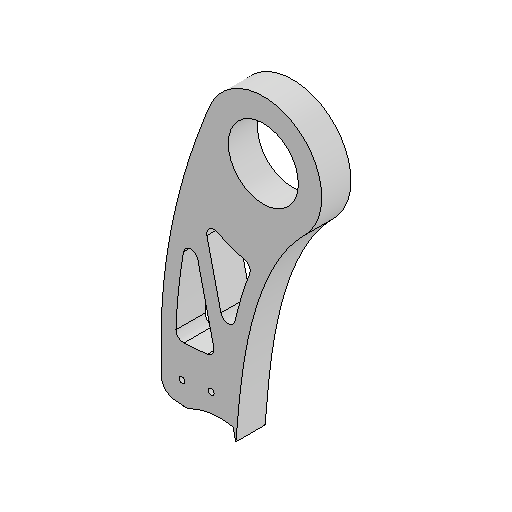
# Autodesk Inventor part: driveshaftsupport_A
Saved by Autodesk Inventor 2025 (Build 290162000, 162)
## iProperties
Created: 2023-03-01
Part Number: driveshaftsupport_A
Material: Generic
Document SubType Name: Modeling
Designer: ralph
Density: 1 g/cm^3
Appearance: Default
Author: ralph
Autodesk Inventor part; units mm, degrees
(part 1 of 2)
ref_plane "YZ Plane" through (0, 0, 0) normal (1, 0, 0) x (0, 1, 0)
ref_plane "XZ Plane" through (0, 0, 0) normal (0, 1, 0) x (-1, 0, 0)
ref_plane "XY Plane" through (0, 0, 0) normal (0, 0, 1) x (1, 0, 0)
ref_plane "Work Plane1" through (0, 0, 0) normal (0, 0, 1) x (1, 0, 0)
sketch "Sketch1" plane through (0, 0, 0) normal (0, 0, 1) x (1, 0, 0)
  arc A0 (-20.648, -102.4649) -> (-16.3515, -107.2084) centre (-14.4346, -101.1546) ccw
  arc A1 (-10.9828, -109.2489) -> (-16.3515, -107.2084) centre (-31.6865, -155.6385) ccw
  arc A2 (-10.9828, -109.2489) -> (-4.2979, -108.3017) centre (-8.3948, -103.4502) ccw
  arc A3 (0.8876, -104.599) -> (-4.2979, -108.3017) centre (21.0506, -138.319) ccw
  arc A4 (7.2668, -104.5186) -> (0.8876, -104.599) centre (4.1465, -110.049) ccw
  arc A5 (7.2668, -104.5186) -> (24.5776, -101.9869) centre (14.2875, -92.075) ccw
  arc A6 (30.7127, -100.2372) -> (24.5776, -101.9869) centre (29.151, -106.3922) ccw
  arc A7 (43.0033, -105.7359) -> (30.7127, -100.2372) centre (21.0506, -138.319) ccw
  arc A8 (43.0033, -105.7359) -> (57.752, -89.4091) centre (49.2125, -96.52) ccw
  arc A9 (57.752, -7.1109) -> (57.752, -89.4091) centre (107.1678, -48.26) ccw
  arc A10 (57.752, -7.1109) -> (57.752, 7.1109) centre (49.2125, 0) ccw
  arc A11 (57.752, 89.4091) -> (57.752, 7.1109) centre (107.1678, 48.26) ccw
  arc A12 (57.752, 89.4091) -> (46.7209, 107.3496) centre (49.2125, 96.52) ccw
  arc A13 (37.2777, 118.8104) -> (46.7209, 107.3496) centre (44.8601, 115.4372) ccw
  arc A14 (37.2777, 118.8104) -> (27.7131, 132.1679) centre (28.575, 122.682) ccw
  arc A15 (-1.8719, 154.7102) -> (27.7131, 132.1679) centre (25.2222, 159.584) ccw
  arc A16 (-1.8719, 154.7102) -> (-9.0898, 161.7077) centre (-11.1125, 152.4) ccw
  arc A17 (-57.3497, 188.5663) -> (-9.0898, 161.7077) centre (11.1567, 254.8735) ccw
  arc A18 (-57.3497, 188.5663) -> (-61.9125, 190.5) centre (-61.9125, 184.15) ccw
  line L0 (-61.9125, -74.837) -> (-61.9125, 190.5)
  arc A19 (-57.4675, -76.6522) -> (-61.9125, -74.837) centre (-61.9125, -81.187) ccw
  arc A20 (-57.4675, -76.6522) -> (-50.3955, -79.3664) centre (-50.8, -69.85) ccw
  arc A21 (-20.648, -102.4649) -> (-50.3955, -79.3664) centre (-49.1581, -108.4774) ccw
  line L1 (-54.9779, 170.3652) -> (-48.8256, 159.5987)
  arc A22 (-48.8539, 153.2488) -> (-48.8256, 159.5987) centre (-54.339, 156.4482) ccw
  arc A23 (-48.8539, 153.2488) -> (-49.1732, 139.4288) centre (-36.5125, 146.05) ccw
  arc A24 (-49.4382, 133.0844) -> (-49.1732, 139.4288) centre (-54.8001, 136.4861) ccw
  line L2 (-49.4382, 133.0844) -> (-55.0158, 124.2927)
  arc A25 (-57.9437, 125.1431) -> (-55.0158, 124.2927) centre (-56.3562, 125.1431) ccw
  line L3 (-57.9437, 125.1431) -> (-57.9437, 169.5776)
  arc A26 (-54.9779, 170.3652) -> (-57.9437, 169.5776) centre (-56.3562, 169.5776) ccw
  line L4 (-57.9437, 16.3803) -> (-57.9437, 88.2093)
  arc A27 (-48.4371, 93.7191) -> (-57.9437, 88.2093) centre (-51.5937, 88.2093) ccw
  line L5 (-48.4371, 93.7191) -> (25.1122, 51.5817)
  arc A28 (24.9048, 45.9631) -> (25.1122, 51.5817) centre (23.5339, 48.8268) ccw
  line L6 (24.9048, 45.9631) -> (-48.8518, 10.6528)
  arc A29 (-57.9437, 16.3803) -> (-48.8518, 10.6528) centre (-51.5937, 16.3803) ccw
  line L7 (-12.5571, -63.0775) -> (-11.8021, -62.3567)
  arc A30 (-6.8531, -63.0782) -> (-11.8021, -62.3567) centre (-9.6098, -64.6534) ccw
  line L8 (-6.8531, -63.0782) -> (0.9035, -76.6523)
  arc A31 (-1.2505, -78.8251) -> (0.9035, -76.6523) centre (-0.4748, -77.44) ccw
  line L9 (-1.2505, -78.8251) -> (-11.2752, -73.2112)
  arc A32 (-12.5571, -63.0775) -> (-11.2752, -73.2112) centre (-8.1726, -67.6708) ccw
  line L10 (8.063, -43.7132) -> (40.1759, -13.8303)
  arc A33 (42.6746, -15.7078) -> (40.1759, -13.8303) centre (41.2574, -14.9925) ccw
  arc A34 (42.6746, -15.7078) -> (35.0956, -43.2986) centre (107.1678, -48.26) ccw
  arc A35 (28.7606, -49.2125) -> (35.0956, -43.2986) centre (28.7606, -42.8625) ccw
  line L11 (28.7606, -49.2125) -> (10.2259, -49.2125)
  arc A36 (8.063, -43.7132) -> (10.2259, -49.2125) centre (10.2259, -46.0375) ccw
  arc A37 (0.0566, -90.8047) -> (0.0035, -91.7596) centre (14.2875, -92.075) ccw
  arc A38 (-5.1562, -94.1671) -> (0.0035, -91.7596) centre (-3.1707, -91.6895) ccw
  arc A39 (-5.1562, -94.1671) -> (-8.4369, -92.4585) centre (-11.1125, -101.6) ccw
  arc A40 (-12.4439, -88.97) -> (-8.4369, -92.4585) centre (-6.6532, -86.3642) ccw
  line L12 (-12.4439, -88.97) -> (-14.871, -83.5766)
  arc A41 (-12.6476, -81.54) -> (-14.871, -83.5766) centre (-13.4233, -82.9251) ccw
  line L13 (-12.6476, -81.54) -> (-1.5545, -87.7521)
  arc A42 (0.0566, -90.8047) -> (-1.5545, -87.7521) centre (-3.1058, -90.5224) ccw
  line L14 (35.1248, 3.9688) -> (-30.4467, 3.9688)
  arc A43 (-31.8177, 10.0075) -> (-30.4467, 3.9688) centre (-30.4467, 7.1438) ccw
  line L15 (-31.8177, 10.0075) -> (27.4027, 38.3586)
  arc A44 (36.3678, 33.8939) -> (27.4027, 38.3586) centre (30.1446, 32.6312) ccw
  arc A45 (36.3678, 33.8939) -> (42.7868, 15.4863) centre (107.1678, 48.26) ccw
  arc A46 (41.5223, 8.0217) -> (42.7868, 15.4863) centre (37.1279, 12.6056) ccw
  arc A47 (41.5223, 8.0217) -> (40.2476, 6.5665) centre (49.2125, 0) ccw
  arc A48 (35.1248, 3.9688) -> (40.2476, 6.5665) centre (35.1248, 10.3188) ccw
  line L16 (-30.2893, 128.8322) -> (-21.4237, 114.8579)
  arc A49 (-24.1047, 109.982) -> (-21.4237, 114.8579) centre (-24.1047, 113.157) ccw
  line L17 (-24.1047, 109.982) -> (-43.146, 109.982)
  arc A50 (-48.5079, 119.7337) -> (-43.146, 109.982) centre (-43.146, 116.332) ccw
  line L18 (-48.5079, 119.7337) -> (-42.7357, 128.8322)
  arc A51 (-37.1087, 131.7749) -> (-42.7357, 128.8322) centre (-37.3737, 125.4305) ccw
  arc A52 (-37.1087, 131.7749) -> (-35.9163, 131.7749) centre (-36.5125, 146.05) ccw
  arc A53 (-30.2893, 128.8322) -> (-35.9163, 131.7749) centre (-35.6513, 125.4305) ccw
  arc A54 (-26.2357, 155.9757) -> (-36.4489, 160.3374) centre (-36.5125, 146.05) ccw
  arc A55 (-41.934, 163.5368) -> (-36.4489, 160.3374) centre (-36.4206, 166.6873) ccw
  line L19 (-41.934, 163.5368) -> (-43.2662, 165.8683)
  arc A56 (-41.0698, 168.0164) -> (-43.2662, 165.8683) centre (-41.8879, 166.6559) ccw
  arc A57 (-41.0698, 168.0164) -> (-20.6642, 158.6488) centre (11.1567, 254.8735) ccw
  arc A58 (-19.7269, 156.4642) -> (-20.6642, 158.6488) centre (-21.1626, 157.1416) ccw
  arc A59 (-19.7269, 156.4642) -> (-20.2275, 155.1645) centre (-11.1125, 152.4) ccw
  arc A60 (-21.7728, 154.038) -> (-20.2275, 155.1645) centre (-21.7467, 155.6253) ccw
  arc A61 (-26.2357, 155.9757) -> (-21.7728, 154.038) centre (-21.6682, 160.3871) ccw
  arc A62 (39.7212, 90.7404) -> (41.5223, 88.4983) centre (49.2125, 96.52) ccw
  arc A63 (42.7868, 81.0337) -> (41.5223, 88.4983) centre (37.1279, 83.9144) ccw
  arc A64 (42.7868, 81.0337) -> (36.5882, 63.6726) centre (107.1678, 48.26) ccw
  arc A65 (27.2278, 59.5175) -> (36.5882, 63.6726) centre (30.3844, 65.0273) ccw
  line L20 (27.2278, 59.5175) -> (-38.1265, 96.9599)
  arc A66 (-37.2022, 99.9191) -> (-38.1265, 96.9599) centre (-37.3374, 98.3373) ccw
  line L21 (-37.2022, 99.9191) -> (34.8381, 93.7648)
  arc A67 (39.7212, 90.7404) -> (34.8381, 93.7648) centre (34.2976, 87.4378) ccw
  line L22 (-57.9437, -42.8625) -> (-57.9437, -24.653)
  arc A68 (-47.137, -20.1298) -> (-57.9437, -24.653) centre (-51.5937, -24.653) ccw
  line L23 (-47.137, -20.1298) -> (-23.138, -43.7759)
  arc A69 (-25.3663, -49.2125) -> (-23.138, -43.7759) centre (-25.3663, -46.0375) ccw
  line L24 (-25.3663, -49.2125) -> (-51.5937, -49.2125)
  arc A70 (-57.9437, -42.8625) -> (-51.5937, -49.2125) centre (-51.5937, -42.8625) ccw
  arc A71 (33.2333, -92.6915) -> (32.5694, -92.5194) centre (21.0506, -138.319) ccw
  arc A72 (28.0165, -88.1193) -> (32.5694, -92.5194) centre (34.1183, -86.3612) ccw
  arc A73 (28.0165, -88.1193) -> (26.6289, -84.8762) centre (14.2875, -92.075) ccw
  arc A74 (26.6006, -78.5263) -> (26.6289, -84.8762) centre (32.114, -81.6768) ccw
  line L25 (26.6006, -78.5263) -> (34.1483, -65.3178)
  arc A75 (37.0671, -65.7217) -> (34.1483, -65.3178) centre (35.5267, -66.1055) ccw
  arc A76 (37.0671, -65.7217) -> (42.7868, -81.0337) centre (107.1678, -48.26) ccw
  arc A77 (41.5223, -88.4983) -> (42.7868, -81.0337) centre (37.1279, -83.9144) ccw
  arc A78 (41.5223, -88.4983) -> (40.0864, -90.1796) centre (49.2125, -96.52) ccw
  arc A79 (33.2333, -92.6915) -> (40.0864, -90.1796) centre (34.8714, -86.5564) ccw
  line L26 (26.9592, -61.9002) -> (19.8008, -74.4274)
  arc A80 (8.7742, -74.4274) -> (19.8008, -74.4274) centre (14.2875, -71.2769) ccw
  line L27 (8.7742, -74.4274) -> (4.3302, -66.6505)
  arc A81 (9.8436, -57.15) -> (4.3302, -66.6505) centre (9.8436, -63.5) ccw
  line L28 (9.8436, -57.15) -> (24.2025, -57.15)
  arc A82 (26.9592, -61.9002) -> (24.2025, -57.15) centre (24.2025, -60.325) ccw
  line L29 (-36.7375, -3.9687) -> (31.0491, -3.9688)
  arc A83 (33.212, -9.4681) -> (31.0491, -3.9688) centre (31.0491, -7.1437) ccw
  line L30 (33.212, -9.4681) -> (-3.4078, -43.5448)
  arc A84 (-12.1903, -43.4194) -> (-3.4078, -43.5448) centre (-7.7336, -38.8962) ccw
  line L31 (-12.1903, -43.4194) -> (-41.1943, -14.842)
  arc A85 (-36.7375, -3.9687) -> (-41.1943, -14.842) centre (-36.7375, -10.3187) ccw
  arc A86 (-23.8518, 139.4288) -> (-22.4829, 143.3475) centre (-36.5125, 146.05) ccw
  arc A87 (-17.3021, 145.1602) -> (-22.4829, 143.3475) centre (-19.3652, 142.7469) ccw
  arc A88 (-17.3021, 145.1602) -> (-16.4703, 144.5248) centre (-11.1125, 152.4) ccw
  arc A89 (-15.0812, 141.8997) -> (-16.4703, 144.5248) centre (-18.2562, 141.8997) ccw
  line L32 (-15.0812, 141.8997) -> (-15.0812, 125.1431)
  arc A90 (-18.0092, 124.2927) -> (-15.0812, 125.1431) centre (-16.6687, 125.1431) ccw
  line L33 (-18.0092, 124.2927) -> (-23.5868, 133.0844)
  arc A91 (-23.8518, 139.4288) -> (-23.5868, 133.0844) centre (-18.2249, 136.4861) ccw
  circle A92 centre (-11.1125, -101.6) radius 3.175
  circle A93 centre (-11.1125, 152.4) radius 3.175
  circle A94 centre (-50.8, -69.85) radius 3.175
  circle A95 centre (-36.5125, 146.05) radius 7.9375
  circle A96 centre (14.2875, -92.075) radius 7.9375
  circle A97 centre (49.2125, 96.52) radius 3.175
  circle A98 centre (49.2125, 0) radius 3.175
  circle A99 centre (49.2125, -96.52) radius 3.175
  circle A100 centre (3.175, 122.682) radius 3.175
  circle A101 centre (-25.4, -69.85) radius 3.175
  circle A102 centre (28.575, 122.682) radius 3.175
  circle A103 centre (-17.4625, 279.4) radius 15.9004
  circle A104 centre (6.6997, 203.792) radius 13.97
  arc A105 (-21.0789, 185.9407) -> (-20.5213, 185.1014) centre (6.6997, 203.792) ccw
  arc A106 (-20.5213, 185.1014) -> (-17.7421, 186.0963) centre (-23.3828, 197.4749) ccw
  arc A107 (-17.7421, 186.0963) -> (-16.917, 185.0092) centre (6.6997, 203.792) ccw
  arc A108 (-16.917, 185.0092) -> (-18.6225, 182.5999) centre (-7.4744, 176.5163) ccw
  arc A109 (-18.6225, 182.5999) -> (-17.9641, 181.8371) centre (6.6997, 203.792) ccw
  arc A110 (-17.9641, 181.8371) -> (-15.3315, 183.1724) centre (-22.3539, 193.7543) ccw
  arc A111 (-15.3315, 183.1724) -> (-14.3766, 182.1973) centre (6.6997, 203.792) ccw
  arc A112 (-14.3766, 182.1973) -> (-15.7668, 179.5933) centre (-3.9441, 174.9549) ccw
  arc A113 (-15.7668, 179.5933) -> (-15.018, 178.919) centre (6.6997, 203.792) ccw
  arc A114 (-15.018, 178.919) -> (-12.5735, 180.5738) centre (-20.8667, 190.1921) ccw
  arc A115 (-12.5735, 180.5738) -> (-11.5039, 179.726) centre (6.6997, 203.792) ccw
  arc A116 (-11.5039, 179.726) -> (-12.5567, 176.9683) centre (-0.246, 173.8483) ccw
  arc A117 (-12.5567, 176.9683) -> (-11.7293, 176.3932) centre (6.6997, 203.792) ccw
  arc A118 (-11.7293, 176.3932) -> (-9.5115, 178.3413) centre (-18.9448, 186.8443) ccw
  arc A119 (-9.5115, 178.3413) -> (-8.3441, 177.6343) centre (6.6997, 203.792) ccw
  arc A120 (-8.3441, 177.6343) -> (-9.043, 174.7663) centre (3.5618, 173.2139) ccw
  arc A121 (-9.043, 174.7663) -> (-8.15, 174.2995) centre (6.6997, 203.792) ccw
  arc A122 (-8.15, 174.2995) -> (-6.1939, 176.5101) centre (-16.6185, 183.7639) ccw
  arc A123 (-6.1939, 176.5101) -> (-4.9471, 175.955) centre (6.6997, 203.792) ccw
  arc A124 (-4.9471, 175.955) -> (-5.281, 173.0221) centre (7.4189, 173.0617) ccw
  arc A125 (-5.281, 173.0221) -> (-4.3365, 172.6709) centre (6.6997, 203.792) ccw
  arc A126 (-4.3365, 172.6709) -> (-2.6729, 175.1093) centre (-13.9245, 180.9992) ccw
  arc A127 (-2.6729, 175.1093) -> (-1.3663, 174.7148) centre (6.6997, 203.792) ccw
  arc A128 (-1.3663, 174.7148) -> (-1.33, 171.7632) centre (11.2648, 173.3941) ccw
  arc A129 (-1.33, 171.7632) -> (-0.349, 171.5331) centre (6.6997, 203.792) ccw
  arc A130 (-0.349, 171.5331) -> (0.9959, 174.1607) centre (-10.9052, 178.5941) ccw
  arc A131 (0.9959, 174.1607) -> (2.3416, 173.9331) centre (6.6997, 203.792) ccw
  arc A132 (2.3416, 173.9331) -> (2.7476, 171.0093) centre (15.0387, 174.206) ccw
  arc A133 (2.7476, 171.0093) -> (3.7497, 170.904) centre (6.6997, 203.792) ccw
  arc A134 (3.7497, 170.904) -> (4.7547, 173.6795) centre (-7.6082, 176.5863) ccw
  arc A135 (4.7547, 173.6795) -> (6.1183, 173.6224) centre (6.6997, 203.792) ccw
  arc A136 (6.1183, 173.6224) -> (6.8875, 170.7725) centre (18.681, 175.4844) ccw
  arc A137 (6.8875, 170.7725) -> (7.8949, 170.7936) centre (6.6997, 203.792) ccw
  arc A138 (7.8949, 170.7936) -> (8.5441, 173.6732) centre (-4.0856, 175.0075) ccw
  arc A139 (8.5441, 173.6732) -> (9.9041, 173.7874) centre (6.6997, 203.792) ccw
  arc A140 (9.9041, 173.7874) -> (11.0244, 171.0564) centre (22.1344, 177.2093) ccw
  arc A141 (11.0244, 171.0564) -> (12.0213, 171.2036) centre (6.6997, 203.792) ccw
  arc A142 (12.0213, 171.2036) -> (12.3044, 174.1418) centre (-0.3929, 173.8827) ccw
  arc A143 (12.3044, 174.1418) -> (13.6394, 174.4256) centre (6.6997, 203.792) ccw
  arc A144 (13.6394, 174.4256) -> (15.0932, 171.8565) centre (25.3444, 179.3534) ccw
  arc A145 (15.0932, 171.8565) -> (16.0637, 172.1275) centre (6.6997, 203.792) ccw
  arc A146 (16.0637, 172.1275) -> (15.9764, 175.0781) centre (3.4116, 173.2296) ccw
  arc A147 (15.9764, 175.0781) -> (17.2653, 175.5269) centre (6.6997, 203.792) ccw
  arc A148 (17.2653, 175.5269) -> (19.0296, 173.1603) centre (28.2603, 181.8829) ccw
  arc A149 (19.0296, 173.1603) -> (19.9585, 173.5508) centre (6.6997, 203.792) ccw
  arc A150 (19.9585, 173.5508) -> (19.502, 176.4672) centre (7.268, 173.0585) ccw
  arc A151 (19.502, 176.4672) -> (20.7245, 177.074) centre (6.6997, 203.792) ccw
  arc A152 (20.7245, 177.074) -> (22.7715, 174.9472) centre (30.8363, 184.7579) ccw
  arc A153 (22.7715, 174.9472) -> (23.6442, 175.451) centre (6.6997, 203.792) ccw
  arc A154 (23.6442, 175.451) -> (22.8258, 178.2872) centre (11.1155, 173.3721) ccw
  arc A155 (22.8258, 178.2872) -> (23.9626, 179.0424) centre (6.6997, 203.792) ccw
  arc A156 (23.9626, 179.0424) -> (26.26, 177.189) centre (33.0315, 187.9331) ccw
  arc A157 (26.26, 177.189) -> (27.0626, 177.7982) centre (6.6997, 203.792) ccw
  arc A158 (27.0626, 177.7982) -> (25.8952, 180.5094) centre (14.8933, 174.1654) ccw
  arc A159 (25.8952, 180.5094) -> (26.9284, 181.4012) centre (6.6997, 203.792) ccw
  arc A160 (26.9284, 181.4012) -> (29.44, 179.8503) centre (34.8116, 191.3584) ccw
  arc A161 (29.44, 179.8503) -> (30.1599, 180.5553) centre (6.6997, 203.792) ccw
  arc A162 (30.1599, 180.5553) -> (28.6619, 183.0989) centre (18.5419, 175.4259) ccw
  arc A163 (28.6619, 183.0989) -> (29.5752, 184.1131) centre (6.6997, 203.792) ccw
  arc A164 (29.5752, 184.1131) -> (32.2613, 182.8892) centre (36.1482, 194.9798) ccw
  arc A165 (32.2613, 182.8892) -> (32.8872, 183.6789) centre (6.6997, 203.792) ccw
  arc A166 (32.8872, 183.6789) -> (31.0823, 186.0146) centre (22.0037, 177.1338) ccw
  arc A167 (31.0823, 186.0146) -> (31.8612, 187.1353) centre (6.6997, 203.792) ccw
  arc A168 (31.8612, 187.1353) -> (34.6796, 186.2577) centre (37.0205, 198.7401) ccw
  arc A169 (34.6796, 186.2577) -> (35.2016, 187.1197) centre (6.6997, 203.792) ccw
  arc A170 (35.2016, 187.1197) -> (33.1181, 189.2107) centre (25.2242, 179.2621) ccw
  arc A171 (33.1181, 189.2107) -> (33.7504, 190.4202) centre (6.6997, 203.792) ccw
  arc A172 (33.7504, 190.4202) -> (36.6566, 189.9028) centre (37.4145, 202.5802) ccw
  arc A173 (36.6566, 189.9028) -> (37.0664, 190.8233) centre (6.6997, 203.792) ccw
  arc A174 (37.0664, 190.8233) -> (34.7373, 192.6368) centre (28.1525, 181.7773) ccw
  arc A175 (34.7373, 192.6368) -> (35.2131, 193.916) centre (6.6997, 203.792) ccw
  arc A176 (35.2131, 193.916) -> (38.1611, 193.7669) centre (37.3242, 206.4393) ccw
  arc A177 (38.1611, 193.7669) -> (38.4524, 194.7316) centre (6.6997, 203.792) ccw
  arc A178 (38.4524, 194.7316) -> (35.9143, 196.2388) centre (30.7425, 184.6396) ccw
  arc A179 (35.9143, 196.2388) -> (36.226, 197.5675) centre (6.6997, 203.792) ccw
  arc A180 (36.226, 197.5675) -> (39.1695, 197.7891) centre (36.7509, 210.2567) ccw
  arc A181 (39.1695, 197.7891) -> (39.3376, 198.7827) centre (6.6997, 203.792) ccw
  arc A182 (39.3376, 198.7827) -> (36.6306, 199.9599) centre (32.9533, 187.804) ccw
  arc A183 (36.6306, 199.9599) -> (36.7733, 201.3172) centre (6.6997, 203.792) ccw
  arc A184 (36.7733, 201.3172) -> (39.6658, 201.906) centre (35.7037, 213.9721) ccw
  arc A185 (39.6658, 201.906) -> (39.708, 202.9128) centre (6.6997, 203.792) ccw
  arc A186 (39.708, 202.9128) -> (36.8749, 203.7415) centre (34.7502, 191.2205) ccw
  arc A187 (36.8749, 203.7415) -> (36.8463, 205.106) centre (6.6997, 203.792) ccw
  arc A188 (36.8463, 205.106) -> (39.6423, 206.0526) centre (34.1991, 217.527) ccw
  arc A189 (39.6423, 206.0526) -> (39.558, 207.0567) centre (6.6997, 203.792) ccw
  arc A190 (39.558, 207.0567) -> (36.6433, 207.5238) centre (36.1046, 194.8353) ccw
  arc A191 (36.6433, 207.5238) -> (36.4439, 208.874) centre (6.6997, 203.792) ccw
  arc A192 (36.4439, 208.874) -> (39.0992, 210.1636) centre (32.2608, 220.8653) ccw
  arc A193 (39.0992, 210.1636) -> (38.8897, 211.1492) centre (6.6997, 203.792) ccw
  arc A194 (38.8897, 211.1492) -> (35.9394, 211.2473) centre (36.9953, 198.5913) ccw
  arc A195 (35.9394, 211.2473) -> (35.5724, 212.5618) centre (6.6997, 203.792) ccw
  arc A196 (35.5724, 212.5618) -> (38.0451, 214.1741) centre (29.9194, 223.9343) ccw
  arc A197 (38.0451, 214.1741) -> (37.7137, 215.1257) centre (6.6997, 203.792) ccw
  arc A198 (37.7137, 215.1257) -> (34.7745, 214.8533) centre (37.4082, 202.4293) ccw
  arc A199 (34.7745, 214.8533) -> (34.2456, 216.1114) centre (6.6997, 203.792) ccw
  arc A200 (34.2456, 216.1114) -> (36.4967, 218.0208) centre (27.2118, 226.6857) ccw
  arc A201 (36.4967, 218.0208) -> (36.0487, 218.9234) centre (6.6997, 203.792) ccw
  arc A202 (36.0487, 218.9234) -> (33.1668, 218.2847) centre (37.3369, 206.2889) ccw
  arc A203 (33.1668, 218.2847) -> (32.4844, 219.4667) centre (6.6997, 203.792) ccw
  arc A204 (32.4844, 219.4667) -> (34.4784, 221.6432) centre (24.1807, 229.076) ccw
  arc A205 (34.4784, 221.6432) -> (33.9208, 222.4825) centre (6.6997, 203.792) ccw
  arc A206 (33.9208, 222.4825) -> (31.1416, 221.4876) centre (36.7823, 210.109) ccw
  arc A207 (31.1416, 221.4876) -> (30.3165, 222.5747) centre (6.6997, 203.792) ccw
  arc A208 (30.3165, 222.5747) -> (32.022, 224.984) centre (20.8739, 231.0676) ccw
  arc A209 (32.022, 224.984) -> (31.3636, 225.7468) centre (6.6997, 203.792) ccw
  arc A210 (31.3636, 225.7468) -> (28.731, 224.4115) centre (35.7534, 213.8296) ccw
  arc A211 (28.731, 224.4115) -> (27.7761, 225.3866) centre (6.6997, 203.792) ccw
  arc A212 (27.7761, 225.3866) -> (29.1663, 227.9906) centre (17.3436, 232.629) ccw
  arc A213 (29.1663, 227.9906) -> (28.4175, 228.6649) centre (6.6997, 203.792) ccw
  arc A214 (28.4175, 228.6649) -> (25.973, 227.0101) centre (34.2662, 217.3918) ccw
  arc A215 (25.973, 227.0101) -> (24.9034, 227.8579) centre (6.6997, 203.792) ccw
  arc A216 (24.9034, 227.8579) -> (25.9562, 230.6156) centre (13.6455, 233.7356) ccw
  arc A217 (25.9562, 230.6156) -> (25.1288, 231.1907) centre (6.6997, 203.792) ccw
  arc A218 (25.1288, 231.1907) -> (22.911, 229.2426) centre (32.3443, 220.7396) ccw
  arc A219 (22.911, 229.2426) -> (21.7436, 229.9496) centre (6.6997, 203.792) ccw
  arc A220 (21.7436, 229.9496) -> (22.4425, 232.8176) centre (9.8377, 234.3701) ccw
  arc A221 (22.4425, 232.8176) -> (21.5495, 233.2844) centre (6.6997, 203.792) ccw
  arc A222 (21.5495, 233.2844) -> (19.5934, 231.0738) centre (30.018, 223.8201) ccw
  arc A223 (19.5934, 231.0738) -> (18.3466, 231.6289) centre (6.6997, 203.792) ccw
  arc A224 (18.3466, 231.6289) -> (18.6805, 234.5618) centre (5.9806, 234.5222) ccw
  arc A225 (18.6805, 234.5618) -> (17.736, 234.913) centre (6.6997, 203.792) ccw
  arc A226 (17.736, 234.913) -> (16.0724, 232.4746) centre (27.324, 226.5847) ccw
  arc A227 (16.0724, 232.4746) -> (14.7658, 232.8691) centre (6.6997, 203.792) ccw
  arc A228 (14.7658, 232.8691) -> (14.7295, 235.8207) centre (2.1347, 234.1898) ccw
  arc A229 (14.7295, 235.8207) -> (13.7485, 236.0508) centre (6.6997, 203.792) ccw
  arc A230 (13.7485, 236.0508) -> (12.4036, 233.4232) centre (24.3047, 228.9899) ccw
  arc A231 (12.4036, 233.4232) -> (11.0579, 233.6508) centre (6.6997, 203.792) ccw
  arc A232 (11.0579, 233.6508) -> (10.6519, 236.5746) centre (-1.6392, 233.3779) ccw
  arc A233 (10.6519, 236.5746) -> (9.6498, 236.6799) centre (6.6997, 203.792) ccw
  arc A234 (9.6498, 236.6799) -> (8.6448, 233.9044) centre (21.0077, 230.9976) ccw
  arc A235 (8.6448, 233.9044) -> (7.2812, 233.9616) centre (6.6997, 203.792) ccw
  arc A236 (7.2812, 233.9616) -> (6.512, 236.8114) centre (-5.2815, 232.0995) ccw
  arc A237 (6.512, 236.8114) -> (5.5046, 236.7903) centre (6.6997, 203.792) ccw
  arc A238 (5.5046, 236.7903) -> (4.8554, 233.9107) centre (17.4851, 232.5764) ccw
  arc A239 (4.8554, 233.9107) -> (3.4954, 233.7965) centre (6.6997, 203.792) ccw
  arc A240 (3.4954, 233.7965) -> (2.3751, 236.5275) centre (-8.7349, 230.3746) ccw
  arc A241 (2.3751, 236.5275) -> (1.3782, 236.3803) centre (6.6997, 203.792) ccw
  arc A242 (1.3782, 236.3803) -> (1.0951, 233.4421) centre (13.7924, 233.7012) ccw
  arc A243 (1.0951, 233.4421) -> (-0.2399, 233.1583) centre (6.6997, 203.792) ccw
  arc A244 (-0.2399, 233.1583) -> (-1.6937, 235.7274) centre (-11.9449, 228.2305) ccw
  arc A245 (-1.6937, 235.7274) -> (-2.6642, 235.4564) centre (6.6997, 203.792) ccw
  arc A246 (-2.6642, 235.4564) -> (-2.5769, 232.5058) centre (9.9879, 234.3543) ccw
  arc A247 (-2.5769, 232.5058) -> (-3.8658, 232.057) centre (6.6997, 203.792) ccw
  arc A248 (-3.8658, 232.057) -> (-5.6301, 234.4236) centre (-14.8608, 225.701) ccw
  arc A249 (-5.6301, 234.4236) -> (-6.559, 234.0331) centre (6.6997, 203.792) ccw
  arc A250 (-6.559, 234.0331) -> (-6.1025, 231.1167) centre (6.1315, 234.5254) ccw
  arc A251 (-6.1025, 231.1167) -> (-7.325, 230.5099) centre (6.6997, 203.792) ccw
  arc A252 (-7.325, 230.5099) -> (-9.372, 232.6367) centre (-17.4368, 222.826) ccw
  arc A253 (-9.372, 232.6367) -> (-10.2447, 232.1329) centre (6.6997, 203.792) ccw
  arc A254 (-10.2447, 232.1329) -> (-9.4263, 229.2967) centre (2.284, 234.2118) ccw
  arc A255 (-9.4263, 229.2967) -> (-10.5631, 228.5415) centre (6.6997, 203.792) ccw
  arc A256 (-10.5631, 228.5415) -> (-12.8605, 230.3949) centre (-19.632, 219.6508) ccw
  arc A257 (-12.8605, 230.3949) -> (-13.6631, 229.7857) centre (6.6997, 203.792) ccw
  arc A258 (-13.6631, 229.7857) -> (-12.4957, 227.0745) centre (-1.4938, 233.4185) ccw
  arc A259 (-12.4957, 227.0745) -> (-13.5289, 226.1827) centre (6.6997, 203.792) ccw
  arc A260 (-13.5289, 226.1827) -> (-16.0405, 227.7336) centre (-21.4121, 216.2255) ccw
  arc A261 (-16.0405, 227.7336) -> (-16.7604, 227.0286) centre (6.6997, 203.792) ccw
  arc A262 (-16.7604, 227.0286) -> (-15.2624, 224.4851) centre (-5.1424, 232.158) ccw
  arc A263 (-15.2624, 224.4851) -> (-16.1757, 223.4708) centre (6.6997, 203.792) ccw
  arc A264 (-16.1757, 223.4708) -> (-18.8618, 224.6947) centre (-22.7487, 212.6041) ccw
  arc A265 (-18.8618, 224.6947) -> (-19.4877, 223.905) centre (6.6997, 203.792) ccw
  arc A266 (-19.4877, 223.905) -> (-17.6828, 221.5693) centre (-8.6042, 230.4501) ccw
  arc A267 (-17.6828, 221.5693) -> (-18.4617, 220.4486) centre (6.6997, 203.792) ccw
  arc A268 (-18.4617, 220.4486) -> (-21.2801, 221.3262) centre (-23.621, 208.8438) ccw
  arc A269 (-21.2801, 221.3262) -> (-21.8021, 220.4643) centre (6.6997, 203.792) ccw
  arc A270 (-21.8021, 220.4643) -> (-19.7186, 218.3732) centre (-11.8247, 228.3218) ccw
  arc A271 (-19.7186, 218.3732) -> (-20.3509, 217.1637) centre (6.6997, 203.792) ccw
  arc A272 (-20.3509, 217.1637) -> (-23.2571, 217.6811) centre (-24.015, 205.0037) ccw
  arc A273 (-23.2571, 217.6811) -> (-23.6669, 216.7606) centre (6.6997, 203.792) ccw
  arc A274 (-23.6669, 216.7606) -> (-21.3378, 214.9471) centre (-14.753, 225.8066) ccw
  arc A275 (-21.3378, 214.9471) -> (-21.8136, 213.6679) centre (6.6997, 203.792) ccw
  arc A276 (-21.8136, 213.6679) -> (-24.7616, 213.817) centre (-23.9247, 201.1446) ccw
  arc A277 (-24.7616, 213.817) -> (-25.0529, 212.8523) centre (6.6997, 203.792) ccw
  arc A278 (-25.0529, 212.8523) -> (-22.5149, 211.3451) centre (-17.343, 222.9443) ccw
  arc A279 (-22.5149, 211.3451) -> (-22.8265, 210.0164) centre (6.6997, 203.792) ccw
  arc A280 (-22.8265, 210.0164) -> (-25.77, 209.7948) centre (-23.3514, 197.3272) ccw
  arc A281 (-25.77, 209.7948) -> (-25.9381, 208.8012) centre (6.6997, 203.792) ccw
  arc A282 (-25.9381, 208.8012) -> (-23.2311, 207.624) centre (-19.5538, 219.7799) ccw
  arc A283 (-23.2311, 207.624) -> (-23.3738, 206.2667) centre (6.6997, 203.792) ccw
  arc A284 (-23.3738, 206.2667) -> (-26.2663, 205.6779) centre (-22.3042, 193.6118) ccw
  arc A285 (-26.2663, 205.6779) -> (-26.3085, 204.6711) centre (6.6997, 203.792) ccw
  arc A286 (-26.3085, 204.6711) -> (-23.4754, 203.8424) centre (-21.3507, 216.3634) ccw
  arc A287 (-23.4754, 203.8424) -> (-23.4468, 202.4779) centre (6.6997, 203.792) ccw
  arc A288 (-23.4468, 202.4779) -> (-26.2428, 201.5313) centre (-20.7996, 190.0569) ccw
  arc A289 (-26.2428, 201.5313) -> (-26.1585, 200.5272) centre (6.6997, 203.792) ccw
  arc A290 (-26.1585, 200.5272) -> (-23.2438, 200.0601) centre (-22.7051, 212.7486) ccw
  arc A291 (-23.2438, 200.0601) -> (-23.0444, 198.7099) centre (6.6997, 203.792) ccw
  arc A292 (-23.0444, 198.7099) -> (-25.6997, 197.4203) centre (-18.8613, 186.7186) ccw
  arc A293 (-25.6997, 197.4203) -> (-25.4902, 196.4347) centre (6.6997, 203.792) ccw
  arc A294 (-25.4902, 196.4347) -> (-22.5399, 196.3366) centre (-23.5958, 208.9926) ccw
  arc A295 (-22.5399, 196.3366) -> (-22.1729, 195.0221) centre (6.6997, 203.792) ccw
  arc A296 (-22.1729, 195.0221) -> (-24.6456, 193.4098) centre (-16.5199, 183.6496) ccw
  arc A297 (-24.6456, 193.4098) -> (-24.3142, 192.4582) centre (6.6997, 203.792) ccw
  arc A298 (-24.3142, 192.4582) -> (-21.375, 192.7307) centre (-24.0087, 205.1546) ccw
  arc A299 (-21.375, 192.7307) -> (-20.8461, 191.4725) centre (6.6997, 203.792) ccw
  arc A300 (-20.8461, 191.4725) -> (-23.0972, 189.5631) centre (-13.8123, 180.8982) ccw
  arc A301 (-23.0972, 189.5631) -> (-22.6492, 188.6605) centre (6.6997, 203.792) ccw
  arc A302 (-22.6492, 188.6605) -> (-19.7673, 189.2992) centre (-23.9374, 201.295) ccw
  arc A303 (-19.7673, 189.2992) -> (-19.0849, 188.1172) centre (6.6997, 203.792) ccw
  arc A304 (-19.0849, 188.1172) -> (-21.0789, 185.9407) centre (-10.7812, 178.5079) ccw
  circle A305 centre (-17.4625, 279.4) radius 25.4
  spline S0 degree 3 poles (-29.446, 168.6111) (-27.6192, 182.9318) (-26.9203, 234.0212) (0.498, 261.4395) knots 0 0 0 0 1 1 1 1
  line L34 (-17.4625, 279.4) -> (0.498, 261.4395) construction
  line L35 (-17.4625, 279.4) -> (7.9375, 279.4) construction
  line L36 (-61.9125, 190.5) -> (-61.9125, 238.0996) construction
  line L37 (-61.9125, 238.0996) -> (-40.9534, 289.0612) construction
  spline S1 degree 2 poles (-61.9125, 190.5) (-61.9125, 238.0996) (-40.9534, 289.0612) knots 1 1 1 2 2 2
  line L38 (-17.4625, 279.4) -> (9.2096, 279.4) construction
  line L39 (-61.9125, 190.5) -> (-61.9125, 171.704)
  line L40 (-61.9125, 171.704) -> (-29.446, 168.6111)
  line L41 (-61.9125, 190.5) -> (-61.9125, 171.704)
  line L42 (-61.9125, 181.102) -> (-28.5539, 177.9242)
  circle A306 centre (-52.7964, 180.2336) radius 3.175
  circle A307 centre (-40.0964, 179.0237) radius 3.175
  arc A308 (-30.8733, 184.5775) -> (-40.0964, 191.7237) centre (-40.0964, 182.1987) ccw
  line L43 (-40.0964, 191.7237) -> (-61.9125, 190.5)
  line L44 (-61.9125, -190.5) -> (-40.0964, -191.7237)
  arc A309 (-40.0964, -191.7237) -> (-30.5714, -182.1987) centre (-40.0964, -182.1987) ccw
  circle A310 centre (-40.0964, -182.1987) radius 2.413
  circle A311 centre (-52.7964, -180.2336) radius 2.413
  ellipse E0 centre (-17.2358, 253.9919) end of major axis (-28.8322, 259.1701) minor radius 12.7
  spline S2 degree 4 poles (-24.0778, 153.0864) (-24.3466, 153.8613) (-24.7111, 154.6089) (-25.1407, 155.336) (-25.6107, 156.0482) knots 0 0 0 0 0 1 1 1 1 1
  spline S3 degree 4 poles (-30.5714, -182.1987) (-30.5714, -172.2165) (-43.0585, -166.7432) (-23.0557, -145.6096) (-13.8897, -132.1844) knots -1 -1 -1 -1 -1 0 0 0 0 0
  arc A312 (7.7524, -112.9699) -> (-13.8897, -132.1844) centre (35.2441, -165.7303) ccw
  arc A313 (15.4566, -109.6241) -> (7.7524, -112.9699) centre (14.2875, -117.475) ccw
  arc A314 (47.014, -107.4129) -> (15.4566, -109.6241) centre (35.2441, -165.7303) ccw
  arc A315 (47.014, -107.4129) -> (57.752, -89.4091) centre (49.2125, -96.52) ccw
  arc A316 (57.752, -7.1109) -> (57.752, -89.4091) centre (107.1678, -48.26) ccw
  arc A317 (57.752, -7.1109) -> (57.752, 7.1109) centre (49.2125, 0) ccw
  arc A318 (57.752, 89.4091) -> (57.752, 7.1109) centre (107.1678, 48.26) ccw
  arc A319 (57.752, 89.4091) -> (46.7209, 107.3496) centre (49.2125, 96.52) ccw
  arc A320 (37.2777, 118.8104) -> (46.7209, 107.3496) centre (44.8601, 115.4372) ccw
  arc A321 (37.2777, 118.8104) -> (26.151, 131.8934) centre (28.575, 122.682) ccw
  arc A322 (-24.0778, 153.0864) -> (26.151, 131.8934) centre (14.7867, 175.0785) ccw
  arc A323 (-27.4024, 160.4437) -> (-25.6107, 156.0482) centre (14.7867, 175.0785) ccw
  arc A324 (-27.4024, 160.4437) -> (-30.8733, 184.5775) centre (-36.5125, 171.45) ccw
  arc A325 (-44.4483, 190.6714) -> (-30.8733, 184.5775) centre (-40.0964, 182.1987) ccw
  spline S4 degree 4 poles (-44.4483, 190.6714) (-44.3174, 190.6481) (-44.1874, 190.6237) (-44.0581, 190.5981) (-43.9297, 190.5715) knots 0 0 0 0 0 1 1 1 1 1
  line L45 (-43.9297, 190.5715) -> (-41.4196, 190.1113)
  arc A326 (-37.5711, 187.788) -> (-41.4196, 190.1113) centre (-42.5646, 183.8654) ccw
  line L46 (-37.5711, 187.788) -> (-35.9517, 185.7265)
  arc A327 (-30.8733, 184.5775) -> (-35.9517, 185.7265) centre (-36.5125, 171.45) ccw
  line L47 (-61.9125, 190.5) -> (-61.9125, -190.5)
  point P0 (0, 0)
  point P1 (-57.9437, 162.8921)
  point P2 (-49.3924, 152.2338)
  point P3 (27.4638, -86.5506)
  point P4 (32.2564, -68.6287)
  point P5 (38.0507, -69.2801)
  point P6 (41.1484, -88.8742)
  point P7 (-4.3192, -67.5126)
  point P8 (-25.8221, 200.765)
  point P9 (-61.9125, 181.102)
  point P10 (-30.5714, 182.1987)
  dimension "d0" = 50.8
  dimension "d1" = 45
  dimension "d3" = 18.796
  dimension "d4" = 6.35
  dimension "d5" = 6.35
  dimension "d6" = 12.7
  dimension "d7" = 9.1161
  constraints: 14 end point, 3 centre point, 3 point on circle, 2 horizontal, 2 midpoint, 2 point on line, 1 coincident, 1 collinear, 1 equal length, 1 parallel, 1 tangent, 9 other
  measures "d0" diameter of A305
  measures "d1" angle of L34 L35
  measures "d3" distance of L0.end L39.end
  measures "d4" diameter of A306
  measures "d5" diameter of A307
  measures "d6" horizontal distance of A307.centre A306.centre
  measures "d7" horizontal distance of point (-61.912, 181.102) A306.centre
extrude "Extrusion1" add sketch "Sketch1" along normal blind 12.7 contours L0 L42 A306 A325 A17 L40 | L0 A18 A17 A306 L42 | A17 A325 L42 S0 | L43 A308 A327 L46 A326 L45 S4 A325 A17 A306 A18 | S1 A305 E0 S0 A269 A270 A272 A273 A274 A276 A277 A278 A280 A281 A282 A284 A285 A286 A288 A289 A290 A324 A308 L43 | A325 L42 A17 | A17 L42 A307 A325 | L42 A325 A324 S0 | A305 E0 A103 | A306 A17 A325 L42 | L42 A325 A17 | A17 A325 S4 L45 A326 L46 A327 L42 A307 | E0 A103 A305 | A305 E0 S0 | A290 A289 A288 S0 | S0 E0 A305 | S0 A270 A269 | A286 A285 A284 S0 | S0 A274 A273 A272 | A282 A281 A280 S0 | S0 A278 A277 A276
sketch "Sketch2" plane through (0, 0, 0) normal (0, 0, -1) x (-1, 0, 0)
  line L0 (36.3108, 151.145) -> (38.286, 150.8307) projected
  line L1 (38.286, 150.8307) -> (38.1088, 149.7177) projected
  arc A0 (36.1337, 150.032) -> (38.1088, 149.7177) centre (36.5125, 146.05) ccw projected
  line L2 (36.1337, 150.032) -> (36.3108, 151.145) projected
  arc A1 (35.8103, 125.4117) -> (36.3775, 122.9364) centre (44.6705, 126.1394) ccw projected
  arc A2 (36.3775, 122.9364) -> (37.6493, 122.964) centre (36.5125, 146.05) ccw projected
  arc A3 (37.6493, 122.964) -> (38.1087, 125.4616) centre (29.2253, 125.8045) ccw projected
  arc A4 (38.1087, 125.4616) -> (39.5067, 125.618) centre (36.5125, 146.05) ccw projected
  arc A5 (39.5067, 125.618) -> (40.5068, 123.2837) centre (48.0946, 127.916) ccw projected
  arc A6 (40.5068, 123.2837) -> (41.7532, 123.538) centre (36.5125, 146.05) ccw projected
  arc A7 (41.7532, 123.538) -> (41.7592, 126.0775) centre (32.9574, 124.8286) ccw projected
  arc A8 (41.7592, 126.0775) -> (43.1068, 126.481) centre (36.5125, 146.05) ccw projected
  arc A9 (43.1068, 126.481) -> (44.5077, 124.3628) centre (51.1464, 130.2755) ccw projected
  arc A10 (44.5077, 124.3628) -> (45.6887, 124.8355) centre (36.5125, 146.05) ccw projected
  arc A11 (45.6887, 124.8355) -> (45.2412, 127.3353) centre (36.8037, 124.5349) ccw projected
  arc A12 (45.2412, 127.3353) -> (46.4951, 127.973) centre (36.5125, 146.05) ccw projected
  arc A13 (46.4951, 127.973) -> (48.2516, 126.1389) centre (53.7278, 133.142) ccw projected
  arc A14 (48.2516, 126.1389) -> (49.3292, 126.8149) centre (36.5125, 146.05) ccw projected
  arc A15 (49.3292, 126.8149) -> (48.4425, 129.1946) centre (40.6407, 124.9326) ccw projected
  arc A16 (48.4425, 129.1946) -> (49.5624, 130.0459) centre (36.5125, 146.05) ccw projected
  arc A17 (49.5624, 130.0459) -> (51.6182, 128.555) centre (55.756, 136.4233) ccw projected
  arc A18 (51.6182, 128.555) -> (52.5578, 129.4125) centre (36.5125, 146.05) ccw projected
  arc A19 (52.5578, 129.4125) -> (51.2605, 131.5956) centre (44.345, 126.0091) ccw projected
  arc A20 (51.2605, 131.5956) -> (52.2103, 132.6333) centre (36.5125, 146.05) ccw projected
  arc A21 (52.2103, 132.6333) -> (54.4993, 131.5334) centre (57.1657, 140.0141) ccw projected
  arc A22 (54.4993, 131.5334) -> (55.2707, 132.5449) centre (36.5125, 146.05) ccw projected
  arc A23 (55.2707, 132.5449) -> (53.6044, 134.4613) centre (47.7976, 127.7298) ccw projected
  arc A24 (53.6044, 134.4613) -> (54.3537, 135.6518) centre (36.5125, 146.05) ccw projected
  arc A25 (54.3537, 135.6518) -> (56.8023, 134.9783) centre (57.9115, 143.7989) ccw projected
  arc A26 (56.8023, 134.9783) -> (57.3806, 136.1113) centre (36.5125, 146.05) ccw projected
  arc A27 (57.3806, 136.1113) -> (55.399, 137.6994) centre (50.8874, 130.0392) ccw projected
  arc A28 (55.399, 137.6994) -> (55.9237, 139.0046) centre (36.5125, 146.05) ccw projected
  arc A29 (55.9237, 139.0046) -> (58.4531, 138.7791) centre (57.9696, 147.656) ccw projected
  arc A30 (58.4531, 138.7791) -> (58.8199, 139.9972) centre (36.5125, 146.05) ccw projected
  arc A31 (58.8199, 139.9972) -> (56.5865, 141.2059) centre (53.5153, 132.8632) ccw projected
  arc A32 (56.5865, 141.2059) -> (56.8697, 142.5838) centre (36.5125, 146.05) ccw projected
  arc A33 (56.8697, 142.5838) -> (59.3988, 142.8136) centre (57.338, 151.4615) ccw projected
  arc A34 (59.3988, 142.8136) -> (59.5422, 144.0776) centre (36.5125, 146.05) ccw projected
  arc A35 (59.5422, 144.0776) -> (57.1288, 144.8681) centre (55.5966, 136.1111) ccw projected
  arc A36 (57.1288, 144.8681) -> (57.1615, 146.2744) centre (36.5125, 146.05) ccw projected
  arc A37 (57.1615, 146.2744) -> (59.6089, 146.9522) centre (56.037, 155.0931) ccw projected
  arc A38 (59.6089, 146.9522) -> (59.5243, 148.2214) centre (36.5125, 146.05) ccw projected
  arc A39 (59.5243, 148.2214) -> (57.0086, 148.5683) centre (57.0646, 139.6785) ccw projected
  arc A40 (57.0086, 148.5683) -> (56.7896, 149.9579) centre (36.5125, 146.05) ccw projected
  arc A41 (56.7896, 149.9579) -> (59.0766, 151.0617) centre (54.1086, 158.434) ccw projected
  arc A42 (59.0766, 151.0617) -> (58.7668, 152.2954) centre (36.5125, 146.05) ccw projected
  arc A43 (58.7668, 152.2954) -> (56.2295, 152.1875) centre (57.872, 143.4506) ccw projected
  arc A44 (56.2295, 152.1875) -> (55.7659, 153.5157) centre (36.5125, 146.05) ccw projected
  arc A45 (55.7659, 153.5157) -> (57.8191, 155.0101) centre (51.6146, 161.3769) ccw projected
  arc A46 (57.8191, 155.0101) -> (57.294, 156.1687) centre (36.5125, 146.05) ccw projected
  arc A47 (57.294, 156.1687) -> (54.8168, 155.6095) centre (57.9929, 147.3062) ccw projected
  arc A48 (54.8168, 155.6095) -> (54.1235, 156.8335) centre (36.5125, 146.05) ccw projected
  arc A49 (54.1235, 156.8335) -> (55.8768, 158.6706) centre (48.6352, 163.8271) ccw projected
  arc A50 (55.8768, 158.6706) -> (55.1532, 159.7168) centre (36.5125, 146.05) ccw projected
  arc A51 (55.1532, 159.7168) -> (52.8157, 158.7242) centre (57.4234, 151.1215) ccw projected
  arc A52 (52.8157, 158.7242) -> (51.915, 159.8048) centre (36.5125, 146.05) ccw projected
  arc A53 (51.915, 159.8048) -> (53.3122, 161.9254) centre (45.2661, 165.706) ccw projected
  arc A54 (53.3122, 161.9254) -> (52.4134, 162.8256) centre (36.5125, 146.05) ccw projected
  arc A55 (52.4134, 162.8256) -> (50.2906, 161.4316) centre (56.1818, 154.7738) ccw projected
  arc A56 (50.2906, 161.4316) -> (49.2114, 162.334) centre (36.5125, 146.05) ccw projected
  arc A57 (49.2114, 162.334) -> (50.2075, 164.67) centre (41.6157, 166.9532) ccw projected
  arc A58 (50.2075, 164.67) -> (49.1624, 165.3952) centre (36.5125, 146.05) ccw projected
  arc A59 (49.1624, 165.3952) -> (47.3227, 163.6446) centre (54.308, 158.1457) ccw projected
  arc A60 (47.3227, 163.6446) -> (46.0998, 164.3398) centre (36.5125, 146.05) ccw projected
  arc A61 (46.0998, 164.3398) -> (46.6627, 166.8161) centre (37.8013, 167.5284) ccw projected
  arc A62 (46.6627, 166.8161) -> (45.5049, 167.343) centre (36.5125, 146.05) ccw projected
  arc A63 (45.5049, 167.343) -> (44.0074, 165.2921) centre (51.8622, 161.1288) ccw projected
  arc A64 (44.0074, 165.2921) -> (42.6799, 165.7577) centre (36.5125, 146.05) ccw projected
  arc A65 (42.6799, 165.7577) -> (42.7917, 168.2948) centre (33.9455, 167.4134) ccw projected
  arc A66 (42.7917, 168.2948) -> (41.5584, 168.6065) centre (36.5125, 146.05) ccw projected
  arc A67 (41.5584, 168.6065) -> (40.4511, 166.3211) centre (48.9231, 163.6273) ccw projected
  arc A68 (40.4511, 166.3211) -> (39.0619, 166.5422) centre (36.5125, 146.05) ccw projected
  arc A69 (39.0619, 166.5422) -> (38.7188, 169.0585) centre (30.1721, 166.6117) ccw projected
  arc A70 (38.7188, 169.0585) -> (37.4497, 169.145) centre (36.5125, 146.05) ccw projected
  arc A71 (37.4497, 169.145) -> (36.7683, 166.6986) centre (45.5852, 165.5608) ccw projected
  arc A72 (36.7683, 166.6986) -> (35.3619, 166.6681) centre (36.5125, 146.05) ccw projected
  arc A73 (35.3619, 166.6681) -> (34.575, 169.0827) centre (26.6026, 165.1492) ccw projected
  arc A74 (34.575, 169.0827) -> (33.3109, 168.9412) centre (36.5125, 146.05) ccw projected
  arc A75 (33.3109, 168.9412) -> (33.0772, 166.4125) centre (41.9556, 166.8672) ccw projected
  arc A76 (33.0772, 166.4125) -> (31.6988, 166.1313) centre (36.5125, 146.05) ccw projected
  arc A77 (31.6988, 166.1313) -> (30.4935, 168.3666) centre (23.3516, 163.0728) ccw projected
  arc A78 (30.4935, 168.3666) -> (29.2749, 168.0016) centre (36.5125, 146.05) ccw projected
  arc A79 (29.2749, 168.0016) -> (29.4966, 165.4718) centre (38.151, 167.5046) ccw projected
  arc A80 (29.4966, 165.4718) -> (28.1905, 164.9491) centre (36.5125, 146.05) ccw projected
  arc A81 (28.1905, 164.9491) -> (26.6055, 166.9332) centre (20.5235, 160.4492) ccw projected
  arc A82 (26.6055, 166.9332) -> (25.4716, 166.3566) centre (36.5125, 146.05) ccw projected
  arc A83 (25.4716, 166.3566) -> (26.1414, 163.907) centre (34.2938, 167.4524) ccw projected
  arc A84 (26.1414, 163.907) -> (24.9497, 163.1594) centre (36.5125, 146.05) ccw projected
  arc A85 (24.9497, 163.1594) -> (23.0359, 164.8286) centre (18.2094, 157.3629) ccw projected
  arc A86 (23.0359, 164.8286) -> (22.0232, 164.0588) centre (36.5125, 146.05) ccw projected
  arc A87 (22.0232, 164.0588) -> (23.1196, 161.7682) centre (30.5079, 166.7123) ccw projected
  arc A88 (23.1196, 161.7682) -> (22.0805, 160.8199) centre (36.5125, 146.05) ccw projected
  arc A89 (22.0805, 160.8199) -> (19.8994, 162.1205) centre (16.4835, 153.9129) ccw projected
  arc A90 (19.8994, 162.1205) -> (19.0404, 161.1822) centre (36.5125, 146.05) ccw projected
  arc A91 (19.0404, 161.1822) -> (20.5282, 159.1242) centre (26.915, 165.3081) ccw projected
  arc A92 (20.5282, 159.1242) -> (19.6752, 158.0056) centre (36.5125, 146.05) ccw projected
  arc A93 (19.6752, 158.0056) -> (17.2969, 158.8959) centre (15.4014, 150.2103) ccw projected
  arc A94 (17.2969, 158.8959) -> (16.6193, 157.8193) centre (36.5125, 146.05) ccw projected
  arc A95 (16.6193, 157.8193) -> (18.4506, 156.06) centre (23.6306, 163.2849) ccw projected
  arc A96 (18.4506, 156.06) -> (17.811, 154.807) centre (36.5125, 146.05) ccw projected
  arc A97 (17.811, 154.807) -> (15.3119, 155.2583) centre (14.9979, 146.3739) ccw projected
  arc A98 (15.3119, 155.2583) -> (14.8375, 154.0781) centre (36.5125, 146.05) ccw projected
  arc A99 (14.8375, 154.0781) -> (16.9535, 152.674) centre (20.7602, 160.7078) ccw projected
  arc A100 (16.9535, 152.674) -> (16.5479, 151.327) centre (36.5125, 146.05) ccw projected
  arc A101 (16.5479, 151.327) -> (14.0084, 151.3248) centre (15.2858, 142.5271) ccw projected
  arc A102 (14.0084, 151.3248) -> (13.7523, 150.0788) centre (36.5125, 146.05) ccw projected
  arc A103 (13.7523, 150.0788) -> (16.0851, 149.0752) centre (18.3961, 157.6595) ccw projected
  arc A104 (16.0851, 149.0752) -> (15.9265, 147.6774) centre (36.5125, 146.05) ccw projected
  arc A105 (15.9265, 147.6774) -> (13.4282, 147.2218) centre (16.2559, 138.7935) ccw projected
  arc A106 (13.4282, 147.2218) -> (13.3987, 145.9501) centre (36.5125, 146.05) ccw projected
  arc A107 (13.3987, 145.9501) -> (15.8732, 145.3791) centre (16.6143, 154.2382) ccw projected
  arc A108 (15.8732, 145.3791) -> (15.9668, 143.9755) centre (36.5125, 146.05) ccw projected
  arc A109 (15.9668, 143.9755) -> (13.59, 143.0811) centre (17.8772, 135.2932) ccw projected
  arc A110 (13.59, 143.0811) -> (13.788, 141.8246) centre (36.5125, 146.05) ccw projected
  arc A111 (13.788, 141.8246) -> (16.3247, 141.7046) centre (15.472, 150.5536) ccw projected
  arc A112 (16.3247, 141.7046) -> (16.6674, 140.3403) centre (36.5125, 146.05) ccw projected
  arc A113 (16.6674, 140.3403) -> (14.4884, 139.0359) centre (20.0973, 132.1386) ccw projected
  arc A114 (14.4884, 139.0359) -> (14.9077, 137.8349) centre (36.5125, 146.05) ccw projected
  arc A115 (14.9077, 137.8349) -> (17.425, 138.1698) centre (15.006, 146.7243) ccw projected
  arc A116 (17.425, 138.1698) -> (18.0058, 136.8885) centre (36.5125, 146.05) ccw projected
  arc A117 (18.0058, 136.8885) -> (16.0948, 135.216) centre (22.8451, 129.4311) ccw projected
  arc A118 (16.0948, 135.216) -> (16.7217, 134.1092) centre (36.5125, 146.05) ccw projected
  arc A119 (16.7217, 134.1092) -> (19.1388, 134.8882) centre (15.2312, 142.8734) ccw projected
  arc A120 (19.1388, 134.8882) -> (19.9391, 133.7313) centre (36.5125, 146.05) ccw projected
  arc A121 (19.9391, 133.7313) -> (18.3574, 131.7444) centre (26.0322, 127.2578) ccw projected
  arc A122 (18.3574, 131.7444) -> (19.1719, 130.7673) centre (36.5125, 146.05) ccw projected
  arc A123 (19.1719, 130.7673) -> (21.411, 131.9654) centre (16.1404, 139.1245) ccw projected
  arc A124 (21.411, 131.9654) -> (22.405, 130.9699) centre (36.5125, 146.05) ccw projected
  arc A125 (22.405, 130.9699) -> (21.2035, 128.7326) centre (29.5561, 125.6884) ccw projected
  arc A126 (21.2035, 128.7326) -> (22.1794, 127.9166) centre (36.5125, 146.05) ccw projected
  arc A127 (22.1794, 127.9166) -> (24.1686, 129.4953) centre (17.7044, 135.5982) ccw projected
  arc A128 (24.1686, 129.4953) -> (25.3244, 128.6933) centre (36.5125, 146.05) ccw projected
  arc A129 (25.3244, 128.6933) -> (24.5417, 126.2774) centre (33.3036, 124.7735) ccw projected
  arc A130 (24.5417, 126.2774) -> (25.6476, 125.6488) centre (36.5125, 146.05) ccw projected
  arc A131 (25.6476, 125.6488) -> (27.323, 127.5572) centre (19.8729, 132.4078) ccw projected
  arc A132 (27.323, 127.5572) -> (28.6033, 126.9745) centre (36.5125, 146.05) ccw projected
  arc A133 (28.6033, 126.9745) -> (28.2646, 124.4577) centre (37.1542, 124.5425) ccw projected
  arc A134 (28.2646, 124.4577) -> (29.465, 124.0366) centre (36.5125, 146.05) ccw projected
  arc A135 (29.465, 124.0366) -> (30.7727, 126.2135) centre (22.5762, 129.656) ccw projected
  arc A136 (30.7727, 126.2135) -> (32.1365, 125.8688) centre (36.5125, 146.05) ccw projected
  arc A137 (32.1365, 125.8688) -> (32.2526, 123.3319) centre (40.9842, 125.0027) ccw projected
  arc A138 (32.2526, 123.3319) -> (33.5089, 123.132) centre (36.5125, 146.05) ccw projected
  arc A139 (33.5089, 123.132) -> (34.4068, 125.5074) centre (25.7274, 127.431) ccw projected
  arc A140 (34.4068, 125.5074) -> (35.8103, 125.4117) centre (36.5125, 146.05) ccw projected
  circle A141 centre (-6.6997, 178.392) radius 13.97 projected
  arc A142 (21.375, 167.3307) -> (24.3142, 167.0582) centre (24.0087, 179.7546) ccw projected
  arc A143 (24.3142, 167.0582) -> (24.6456, 168.0098) centre (-6.6997, 178.392) ccw projected
  arc A144 (24.6456, 168.0098) -> (22.1729, 169.6221) centre (16.5199, 158.2496) ccw projected
  arc A145 (22.1729, 169.6221) -> (22.5399, 170.9366) centre (-6.6997, 178.392) ccw projected
  arc A146 (22.5399, 170.9366) -> (25.4902, 171.0347) centre (23.5958, 183.5926) ccw projected
  arc A147 (25.4902, 171.0347) -> (25.6997, 172.0203) centre (-6.6997, 178.392) ccw projected
  arc A148 (25.6997, 172.0203) -> (23.0444, 173.3099) centre (18.8613, 161.3186) ccw projected
  arc A149 (23.0444, 173.3099) -> (23.2438, 174.6601) centre (-6.6997, 178.392) ccw projected
  arc A150 (23.2438, 174.6601) -> (26.1585, 175.1272) centre (22.7051, 187.3486) ccw projected
  arc A151 (26.1585, 175.1272) -> (26.2428, 176.1313) centre (-6.6997, 178.392) ccw projected
  arc A152 (26.2428, 176.1313) -> (23.4468, 177.0779) centre (20.7996, 164.6569) ccw projected
  arc A153 (23.4468, 177.0779) -> (23.4754, 178.4424) centre (-6.6997, 178.392) ccw projected
  arc A154 (23.4754, 178.4424) -> (26.3085, 179.2711) centre (21.3507, 190.9634) ccw projected
  arc A155 (26.3085, 179.2711) -> (26.2663, 180.2779) centre (-6.6997, 178.392) ccw projected
  arc A156 (26.2663, 180.2779) -> (23.3738, 180.8667) centre (22.3042, 168.2118) ccw projected
  arc A157 (23.3738, 180.8667) -> (23.2311, 182.224) centre (-6.6997, 178.392) ccw projected
  arc A158 (23.2311, 182.224) -> (25.9381, 183.4012) centre (19.5538, 194.3799) ccw projected
  arc A159 (25.9381, 183.4012) -> (25.77, 184.3948) centre (-6.6997, 178.392) ccw projected
  arc A160 (25.77, 184.3948) -> (22.8265, 184.6164) centre (23.3514, 171.9272) ccw projected
  arc A161 (22.8265, 184.6164) -> (22.5149, 185.9451) centre (-6.6997, 178.392) ccw projected
  arc A162 (22.5149, 185.9451) -> (25.0529, 187.4523) centre (17.343, 197.5443) ccw projected
  arc A163 (25.0529, 187.4523) -> (24.7616, 188.417) centre (-6.6997, 178.392) ccw projected
  arc A164 (24.7616, 188.417) -> (21.8136, 188.2679) centre (23.9247, 175.7446) ccw projected
  arc A165 (21.8136, 188.2679) -> (21.3378, 189.5471) centre (-6.6997, 178.392) ccw projected
  arc A166 (21.3378, 189.5471) -> (23.6669, 191.3606) centre (14.753, 200.4066) ccw projected
  arc A167 (23.6669, 191.3606) -> (23.2571, 192.2811) centre (-6.6997, 178.392) ccw projected
  arc A168 (23.2571, 192.2811) -> (20.3509, 191.7637) centre (24.015, 179.6037) ccw projected
  arc A169 (20.3509, 191.7637) -> (19.7186, 192.9732) centre (-6.6997, 178.392) ccw projected
  arc A170 (19.7186, 192.9732) -> (21.8021, 195.0643) centre (11.8247, 202.9218) ccw projected
  arc A171 (21.8021, 195.0643) -> (21.2801, 195.9262) centre (-6.6997, 178.392) ccw projected
  arc A172 (21.2801, 195.9262) -> (18.4617, 195.0486) centre (23.621, 183.4438) ccw projected
  arc A173 (18.4617, 195.0486) -> (17.6828, 196.1693) centre (-6.6997, 178.392) ccw projected
  arc A174 (17.6828, 196.1693) -> (19.4877, 198.505) centre (8.6042, 205.0501) ccw projected
  arc A175 (19.4877, 198.505) -> (18.8618, 199.2947) centre (-6.6997, 178.392) ccw projected
  arc A176 (18.8618, 199.2947) -> (16.1757, 198.0708) centre (22.7487, 187.2041) ccw projected
  arc A177 (16.1757, 198.0708) -> (15.2624, 199.0851) centre (-6.6997, 178.392) ccw projected
  arc A178 (15.2624, 199.0851) -> (16.7604, 201.6286) centre (5.1424, 206.758) ccw projected
  arc A179 (16.7604, 201.6286) -> (16.0405, 202.3336) centre (-6.6997, 178.392) ccw projected
  arc A180 (16.0405, 202.3336) -> (13.5289, 200.7827) centre (21.4121, 190.8255) ccw projected
  arc A181 (13.5289, 200.7827) -> (12.4957, 201.6745) centre (-6.6997, 178.392) ccw projected
  arc A182 (12.4957, 201.6745) -> (13.6631, 204.3857) centre (1.4938, 208.0185) ccw projected
  arc A183 (13.6631, 204.3857) -> (12.8605, 204.9949) centre (-6.6997, 178.392) ccw projected
  arc A184 (12.8605, 204.9949) -> (10.5631, 203.1415) centre (19.632, 194.2508) ccw projected
  arc A185 (10.5631, 203.1415) -> (9.4263, 203.8967) centre (-6.6997, 178.392) ccw projected
  arc A186 (9.4263, 203.8967) -> (10.2447, 206.7329) centre (-2.284, 208.8118) ccw projected
  arc A187 (10.2447, 206.7329) -> (9.372, 207.2367) centre (-6.6997, 178.392) ccw projected
  arc A188 (9.372, 207.2367) -> (7.325, 205.1099) centre (17.4368, 197.426) ccw projected
  arc A189 (7.325, 205.1099) -> (6.1025, 205.7167) centre (-6.6997, 178.392) ccw projected
  arc A190 (6.1025, 205.7167) -> (6.559, 208.6331) centre (-6.1315, 209.1254) ccw projected
  arc A191 (6.559, 208.6331) -> (5.6301, 209.0236) centre (-6.6997, 178.392) ccw projected
  arc A192 (5.6301, 209.0236) -> (3.8658, 206.657) centre (14.8608, 200.301) ccw projected
  arc A193 (3.8658, 206.657) -> (2.5769, 207.1058) centre (-6.6997, 178.392) ccw projected
  arc A194 (2.5769, 207.1058) -> (2.6642, 210.0564) centre (-9.9879, 208.9543) ccw projected
  arc A195 (2.6642, 210.0564) -> (1.6937, 210.3274) centre (-6.6997, 178.392) ccw projected
  arc A196 (1.6937, 210.3274) -> (0.2399, 207.7583) centre (11.9449, 202.8305) ccw projected
  arc A197 (0.2399, 207.7583) -> (-1.0951, 208.0421) centre (-6.6997, 178.392) ccw projected
  arc A198 (-1.0951, 208.0421) -> (-1.3782, 210.9803) centre (-13.7924, 208.3012) ccw projected
  arc A199 (-1.3782, 210.9803) -> (-2.3751, 211.1275) centre (-6.6997, 178.392) ccw projected
  arc A200 (-2.3751, 211.1275) -> (-3.4954, 208.3965) centre (8.7349, 204.9746) ccw projected
  arc A201 (-3.4954, 208.3965) -> (-4.8554, 208.5107) centre (-6.6997, 178.392) ccw projected
  arc A202 (-4.8554, 208.5107) -> (-5.5046, 211.3903) centre (-17.4851, 207.1764) ccw projected
  arc A203 (-5.5046, 211.3903) -> (-6.512, 211.4114) centre (-6.6997, 178.392) ccw projected
  arc A204 (-6.512, 211.4114) -> (-7.2812, 208.5616) centre (5.2815, 206.6995) ccw projected